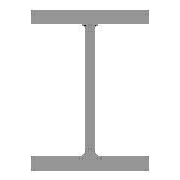
# Autodesk Inventor part: DIN 1025 - IPE 220-1497,05
Saved by Autodesk Inventor 2025 (Build 290162000, 162)
## iProperties
_CCFamilyMember: 80
_CCFamilyDisplayName: DIN 1025-5 IPE - Hot rolled I-beam IPE
_FrameMemberDoc: Frame Member File
_Version: 25.0.0
_GetPNFromCC: 1
Created: 2024-05-05
Part Number: DIN 1025 - IPE 220-1497,05
Material: Steel, Mild
Description: Hot rolled I-beam IPE
Document SubType Name: Modeling
Standard: DIN 1025
Designer: zulet
Standard Revision: 1994
Standards Organization: DIN
Language: en-US
Size Designation: IPE 220
Categories: <MemberInstance><Categories><Category DisplayName="Structural Shapes" InternalName="089c4875-fa83-4c05-b084-43b9cc11f5ed" Mnemonic="GRDR"><CategoryParameter DisplayName="Mass per Length Unit" InternalName="0bb95a10-148f-4027-a459-38d7b056702a" Mnemonic="shpmass"/><CategoryParameter DisplayName="Section Area" InternalName="1ff91680-64b0-4202-b9a3-7fd3f94bba3b" Mnemonic="secarea"/><CategoryParameter DisplayName="Radius of Gyration (x)" InternalName="25778675-03e9-40c1-b6a8-4a9ed693320d" Mnemonic="gyrradx"/><CategoryParameter DisplayName="Torsional Rigidity Modulus" InternalName="26c1ec35-5026-4c63-ad0a-751cf684a536" Mnemonic="torrigmod"/><CategoryParameter DisplayName="Distance of the Center of Gravity X-X" InternalName="26c9bdb8-9c79-4b4f-a92e-8e197583c9c4" Mnemonic="grcendistX"/><CategoryParameter DisplayName="Legacy Member ID" InternalName="340afe4f-75d7-48d3-ab7d-943f3c3da468" Mnemonic="LegacyMemberID"/><CategoryParameter DisplayName="Base Length" InternalName="42e34263-8f20-4d0e-ad48-bf1385b87c24" Mnemonic="shplen"/><CategoryParameter DisplayName="Moment of Inertia (y)" InternalName="4b9f58ea-bced-460e-81ea-3d29ca5a49e3" Mnemonic="inermomy"/><CategoryParameter DisplayName="Moment of Inertia (x)" InternalName="4cd780bc-73d7-43ac-917a-579e5cbd684d" Mnemonic="inermomx"/><CategoryParameter DisplayName="Custom Base Point" InternalName="4f1d1b73-316d-484b-a3df-9cbabb16eb77" Mnemonic="shpBasePoint"/><CategoryParameter DisplayName="Shape Height" InternalName="50274e7d-5ac0-4796-92cb-c59e54983c67" Mnemonic="shpheig"/><CategoryParameter DisplayName="Section Module (y)" InternalName="59eaa5e9-d227-48dc-b6c1-6920f96e0f95" Mnemonic="secmody"/><CategoryParameter DisplayName="Section Designation" InternalName="5a64d034-428d-49c8-ba32-7619764de20f" Mnemonic="shpdes"/><CategoryParameter DisplayName="Section Module (x)" InternalName="72cfad18-cf51-4ed4-aaa7-c6b224f8419f" Mnemonic="secmodx"/><CategoryParameter DisplayName="Torsional Section Modulus" InternalName="7c55a8dc-8844-49f9-a867-cc677b30ec9a" Mnemonic="torsecmod"/><CategoryParameter DisplayName="Shape Width" InternalName="7c717d54-a18f-4666-b4d4-573cce22c62c" Mnemonic="shpwdth"/><CategoryParameter DisplayName="Second Shape Thickness" InternalName="9251a8e1-85fd-4e47-af99-afdb762317d9" Mnemonic="shpthick2"/><CategoryParameter DisplayName="FG Authored" InternalName="9c666724-f362-4ea7-ac62-f6a007de5c69" Mnemonic="shpFGAuto"/><CategoryParameter DisplayName="Distance of the Center of Gravity Y-Y" InternalName="bcc4fb17-7af4-436a-8f8c-d0aa3b0248c5" Mnemonic="grcendistY"/><CategoryParameter DisplayName="Radius of Gyration (y)" InternalName="bfa18ebe-1636-4dbe-8d42-b263e0b73184" Mnemonic="gyrrady"/><CategoryParameter DisplayName="Shape Thickness" InternalName="d109cf76-8eb4-42fc-9800-4409734adc67" Mnemonic="shpthick"/><CategoryParameter DisplayName="Coefficient of Shear Displacement" InternalName="de4c90c6-aaa8-468f-a335-6737b311b5d3" Mnemonic="shdispc"/><Category DisplayName="I-Beams" InternalName="6918ea94-8af8-4304-ae03-7d2c1ce55d4b" Mnemonic="ISHP"><CategoryParameter DisplayName="Mass per Length Unit" InternalName="0dc32564-f4aa-4aa4-8c75-62cb498c92c3" Mnemonic="shpmass"/><CategoryParameter DisplayName="Radius of Gyration (y)" InternalName="0f8afd8f-b9f7-472e-8e75-9212891574fd" Mnemonic="gyrrady"/><CategoryParameter DisplayName="Second Shape Thickness" InternalName="391ebf09-f515-4c94-817f-86f5e53f4689" Mnemonic="shpthick2"/><CategoryParameter DisplayName="Moment of Inertia (x)" InternalName="a758f08a-3b45-4a09-8ee4-ba904e580c14" Mnemonic="inermomx"/><CategoryParameter DisplayName="Moment of Inertia (y)" InternalName="ae881498-39b5-464d-9622-212b1cfb5926" Mnemonic="inermomy"/><CategoryParameter DisplayName="Section Area" InternalName="bf9dd762-a4b6-4f54-802b-8b144141f7fb" Mnemonic="secarea"/><CategoryParameter DisplayName="Section Module (y)" InternalName="c0ad6f84-71f4-4f7a-a8c1-bbe4f36d703a" Mnemonic="secmody"/><CategoryParameter DisplayName="Shape Thickness" InternalName="c729d173-373e-41ba-bff7-d28a079d944c" Mnemonic="shpthick"/><CategoryParameter DisplayName="Radius of Gyration (x)" InternalName="db90017b-4fac-4daa-80b0-a7886743939d" Mnemonic="gyrradx"/><CategoryParameter DisplayName="Section Module (x)" InternalName="e71bf9c5-e82b-494f-914d-abe97254150e" Mnemonic="secmodx"/><CategoryParameter DisplayName="Shape Width" InternalName="f705f81c-b398-4253-aed1-763ae4858594" Mnemonic="shpwdth"/></Category></Category><Category DisplayName="DataType" InternalName="23b78d0f-2648-40c6-8793-ca6db495c9e8" Mnemonic="DATATYPE"><CategoryParameter DisplayName="DisplayName" InternalName="05415f3d-3907-474b-a020-eb9d644f4cf3" Mnemonic="DISPLAYNAME"/><CategoryParameter DisplayName="Standard" InternalName="0c0a119c-1e12-4c84-803f-101930972f5e" Mnemonic="STANDARD"/><CategoryParameter DisplayName="Description" InternalName="13903e3d-64b1-4950-80da-f627842ea37f" Mnemonic="DESCRIPTION"/><CategoryParameter DisplayName="Designation" InternalName="2675968c-4ce5-49e0-a4f5-552d29089031" Mnemonic="DESIGNATION"/><CategoryParameter DisplayName="Default Row" InternalName="2af9ec52-faaa-4026-b378-f9fa4afca842" Mnemonic="DEFAULTROW"/><CategoryParameter DisplayName="Folder Name" InternalName="3f06958e-8713-4116-9be7-ed6184ecc97b" Mnemonic="FOLDERNAME"/><CategoryParameter DisplayName="Revision Guid" InternalName="45a75005-10b1-4dfc-8d6d-dfe629f0b93c" Mnemonic="REVISIONGUID"/><CategoryParameter DisplayName="FileName" InternalName="8b46a4cc-9585-4fed-90c3-899f57e09a73" Mnemonic="FILENAME"/><CategoryParameter DisplayName="StdsOrg" InternalName="8f5914e1-4693-403f-8ab5-d37768198c9d" Mnemonic="STDSORG"/><CategoryParameter DisplayName="Family Version" InternalName="914462f6-6e19-4b14-ba84-155b9680b1d0" Mnemonic="FAMILYREVISION"/><CategoryParameter DisplayName="Standard Revision" InternalName="91d5a463-65c2-4fde-b823-3b7fea5e8e17" Mnemonic="STANDARDREVISION"/><CategoryParameter DisplayName="Member Revision" InternalName="a65d44b9-392f-4f4f-857b-e4b3d54996fe" Mnemonic="MEMBERREVISION"/><CategoryParameter DisplayName="ClipFormat" InternalName="bc51e27b-3422-4e78-93ef-cec197ddf230" Mnemonic="CLIPFORMAT"/><CategoryParameter DisplayName="Manufacturer" InternalName="cd6c7a72-a28a-4e50-99a9-2c7f4e13e5ad" Mnemonic="MANUFACTURER"/><CategoryParameter DisplayName="InternalName" InternalName="cf1d0246-76d9-4b4a-8305-fa0409afb5c1" Mnemonic="INTERNALNAME"/><CategoryParameter DisplayName="IsMetric" InternalName="e2385c5b-1ea4-4823-96a8-8de651266ec3" Mnemonic="ISMETRIC"/><Category DisplayName="Part" InternalName="c0e0b642-3bcb-4cc8-9e80-f96d35c4afa4" Mnemonic="PART"><CategoryParameter DisplayName="Part Number" InternalName="016b6077-bfbe-49bd-92c9-d8d59c39c941" Mnemonic="PARTNUMBER"/><CategoryParameter DisplayName="Stock Number" InternalName="4dba7c1c-e26c-444e-836c-b08b433409a8" Mnemonic="STOCKNUMBER"/><CategoryParameter DisplayName="Material Key" InternalName="5c9a8adb-dd2b-4535-b97f-0a94a95fe41f" Mnemonic="MATERIALKEY"/><CategoryParameter DisplayName="Material" InternalName="818a152a-d3c3-49ca-80ee-df7d91421b8e" Mnemonic="MATERIAL"/></Category></Category><Category DisplayName="LegacyMap" InternalName="cd87c42b-3e48-431e-b5c0-1cbeb14dfe77" Mnemonic="LEGACYMAP"><CategoryParameter DisplayName="unique DA member ID" InternalName="0918ad47-427f-4fed-ae26-24c81c58f590" Mnemonic="DACOOKIE"/><CategoryParameter DisplayName="Merge11 ID" InternalName="0ee8fb18-e2ed-4f39-96f6-1f4b5f50aa71" Mnemonic="MERGE11"/><CategoryParameter DisplayName="unique CC member ID" InternalName="5193edd4-b2b0-4ab4-9d54-de900eee34e0" Mnemonic="CCCOOKIE"/><CategoryParameter DisplayName="Split ID" InternalName="72b5c83c-be7f-45c4-ae51-9160ea6deb26" Mnemonic="SPLIT"/><CategoryParameter DisplayName="MemberID" InternalName="8e5e0294-fc51-4c8f-b3d7-003dc5ed94f6" Mnemonic="MEMBERID"/><CategoryParameter DisplayName="CatalogName" InternalName="d99d1e27-aa94-4de2-af4c-c348882a6f4f" Mnemonic="CATALOGNAME"/><CategoryParameter DisplayName="FamilyNumber" InternalName="e705e1f4-09cb-413e-91f9-551b4188271e" Mnemonic="FAMILYNUMBER"/></Category></Categories><FamilyTemplate Id="D1025_2"><FamilyTemplateParameters><FamilyTemplateParameter ObjectType="kUserParameterObject" ValueType="xs:double" Id="1" ObjectReferenceKey="ParH"/><FamilyTemplateParameter ObjectType="kUserParameterObject" ValueType="xs:double" Id="2" ObjectReferenceKey="b"/><FamilyTemplateParameter ObjectType="kUserParameterObject" ValueType="xs:double" Id="3" ObjectReferenceKey="B_L"/><FamilyTemplateParameter ObjectType="kUserParameterObject" ValueType="xs:double" Id="4" ObjectReferenceKey="t1"/><FamilyTemplateParameter ObjectType="kUserParameterObject" ValueType="xs:double" Id="5" ObjectReferenceKey="t2"/><FamilyTemplateParameter ObjectType="kUserParameterObject" ValueType="xs:double" Id="6" ObjectReferenceKey="R1"/><FamilyTemplateParameter ObjectType="kPropertyObject" ValueType="xs:string" Id="100" ObjectReferenceKey="{32853F0F-3444-11d1-9E93-0060B03C1CA6}" SubObjectId="52"/><FamilyTemplateParameter ObjectType="kPropertyObject" ValueType="xs:string" Id="105" ObjectReferenceKey="{32853F0F-3444-11d1-9E93-0060B03C1CA6}" SubObjectId="5"/><FamilyTemplateParameter ObjectType="kPartComponentDefinitionObject" ValueType="xs:string" Id="110" SubObjectId="Material"/><FamilyTemplateParameter ObjectType="kPropertyObject" ValueType="xs:string" Id="112" ObjectReferenceKey="{32853F0F-3444-11d1-9E93-0060B03C1CA6}" SubObjectId="55"/></FamilyTemplateParameters></FamilyTemplate><CategoryParameterMap><ParamToTemplateMap><ParamToTemplate CategoryParameter="//CategoryParameter[@InternalName='05415f3d-3907-474b-a020-eb9d644f4cf3']" ConstantValue="DIN 1025-5 IPE"/><ParamToTemplate CategoryParameter="//CategoryParameter[@InternalName='cf1d0246-76d9-4b4a-8305-fa0409afb5c1']" ConstantValue="11DEA241-3E29-4894-9654-6C8D07453054"/><ParamToTemplate CategoryParameter="//CategoryParameter[@InternalName='3f06958e-8713-4116-9be7-ed6184ecc97b']" ConstantValue="DIN 1025 IPE"/><ParamToTemplate CategoryParameter="//CategoryParameter[@InternalName='914462f6-6e19-4b14-ba84-155b9680b1d0']" ConstantValue="10"/><ParamToTemplate CategoryParameter="//CategoryParameter[@InternalName='bc51e27b-3422-4e78-93ef-cec197ddf230']" ConstantValue="CF_INVENTOR.STDPARTS"/><ParamToTemplate CategoryParameter="//CategoryParameter[@InternalName='e2385c5b-1ea4-4823-96a8-8de651266ec3']" ConstantValue="true"/><ParamToTemplate CategoryParameter="//CategoryParameter[@InternalName='13903e3d-64b1-4950-80da-f627842ea37f']" ConstantValue="Hot rolled I-beam IPE"/><ParamToTemplate CategoryParameter="//CategoryParameter[@InternalName='8f5914e1-4693-403f-8ab5-d37768198c9d']" ConstantValue="DIN"/><ParamToTemplate CategoryParameter="//CategoryParameter[@InternalName='0c0a119c-1e12-4c84-803f-101930972f5e']" ConstantValue="DIN 1025"/><ParamToTemplate CategoryParameter="//CategoryParameter[@InternalName='cd6c7a72-a28a-4e50-99a9-2c7f4e13e5ad']" TemplateParameter="104"/><ParamToTemplate CategoryParameter="//CategoryParameter[@InternalName='91d5a463-65c2-4fde-b823-3b7fea5e8e17']" ConstantValue="1994"/><ParamToTemplate CategoryParameter="//CategoryParameter[@InternalName='45a75005-10b1-4dfc-8d6d-dfe629f0b93c']" ConstantValue="b36a5bb9-0290-4eb4-bba2-e462c37a096a"/><ParamToTemplate CategoryParameter="//CategoryParameter[@InternalName='2af9ec52-faaa-4026-b378-f9fa4afca842']" ConstantValue="10"/><ParamToTemplate CategoryParameter="//CategoryParameter[@InternalName='9c666724-f362-4ea7-ac62-f6a007de5c69']" ConstantValue="1"/><ParamToTemplate CategoryParameter="//CategoryParameter[@InternalName='8b46a4cc-9585-4fed-90c3-899f57e09a73']" ConstantValue="DIN 1025 - IPE 360-1"/><ParamToTemplate CategoryParameter="//CategoryParameter[@InternalName='a65d44b9-392f-4f4f-857b-e4b3d54996fe']" ConstantValue="2F7BE790-9201-4313-A6B9-FAB6FCE7215E"/><ParamToTemplate CategoryParameter="//CategoryParameter[@InternalName='a758f08a-3b45-4a09-8ee4-ba904e580c14']" ConstantValue="1.627e+008"/><ParamToTemplate CategoryParameter="//CategoryParameter[@InternalName='ae881498-39b5-464d-9622-212b1cfb5926']" ConstantValue="1.04e+007"/><ParamToTemplate CategoryParameter="//CategoryParameter[@InternalName='e71bf9c5-e82b-494f-914d-abe97254150e']" ConstantValue="904000"/><ParamToTemplate CategoryParameter="//CategoryParameter[@InternalName='c0ad6f84-71f4-4f7a-a8c1-bbe4f36d703a']" ConstantValue="123000"/><ParamToTemplate CategoryParameter="//CategoryParameter[@InternalName='bf9dd762-a4b6-4f54-802b-8b144141f7fb']" ConstantValue="7270"/><ParamToTemplate CategoryParameter="//CategoryParameter[@InternalName='7c55a8dc-8844-49f9-a867-cc677b30ec9a']" ConstantValue="29381,034"/><ParamToTemplate CategoryParameter="//CategoryParameter[@InternalName='26c1ec35-5026-4c63-ad0a-751cf684a536']" ConstantValue="373139,13"/><ParamToTemplate CategoryParameter="//CategoryParameter[@InternalName='de4c90c6-aaa8-468f-a335-6737b311b5d3']" ConstantValue="2,1"/><ParamToTemplate CategoryParameter="//CategoryParameter[@InternalName='db90017b-4fac-4daa-80b0-a7886743939d']" ConstantValue="150"/><ParamToTemplate CategoryParameter="//CategoryParameter[@InternalName='0f8afd8f-b9f7-472e-8e75-9212891574fd']" ConstantValue="37,9"/><ParamToTemplate CategoryParameter="//CategoryParameter[@InternalName='0918ad47-427f-4fed-ae26-24c81c58f590']" ConstantValue="*DIN~D1025_5~IPE 360-25000*"/><ParamToTemplate CategoryParameter="//CategoryParameter[@InternalName='0ee8fb18-e2ed-4f39-96f6-1f4b5f50aa71']" ConstantValue="^38b60987-b6a5-40f3-bbfa-fc2af2db0cf9#13^5B1291D4-26CA-46F0-A3B1-56EC9DD4A035#130^"/><ParamToTemplate CategoryParameter="//CategoryParameter[@InternalName='42e34263-8f20-4d0e-ad48-bf1385b87c24']" TemplateParameter="3"/><ParamToTemplate CategoryParameter="//CategoryParameter[@InternalName='2675968c-4ce5-49e0-a4f5-552d29089031']" TemplateParameter="100"/><ParamToTemplate CategoryParameter="//CategoryParameter[@InternalName='818a152a-d3c3-49ca-80ee-df7d91421b8e']" TemplateParameter="110"/><ParamToTemplate CategoryParameter="//CategoryParameter[@InternalName='016b6077-bfbe-49bd-92c9-d8d59c39c941']" TemplateParameter="105"/><ParamToTemplate CategoryParameter="//CategoryParameter[@InternalName='50274e7d-5ac0-4796-92cb-c59e54983c67']" TemplateParameter="1"/><ParamToTemplate CategoryParameter="//CategoryParameter[@InternalName='4dba7c1c-e26c-444e-836c-b08b433409a8']" TemplateParameter="112"/><ParamToTemplate CategoryParameter="//CategoryParameter[@InternalName='f705f81c-b398-4253-aed1-763ae4858594']" TemplateParameter="2"/><ParamToTemplate CategoryParameter="//CategoryParameter[@InternalName='c729d173-373e-41ba-bff7-d28a079d944c']" TemplateParameter="4"/></ParamToTemplateMap></CategoryParameterMap></MemberInstance>
Stock Number: IPE 220
Density: 7.85 g/cm^3
Appearance: Semi-Polished
IsCustomPart: 1
G_L: 1497,050 mm
G_W: 110,000 mm
G_H: 220,000 mm
+E306E2F0-DEFC-4B6E-B958-F0CDA3C58A72+CUTDETAIL1: Miter 45,00 deg
+04264D6A-114A-40A8-9F54-E6A20931D243+CUTDETAIL2: Miter 45,00 deg
+CD89E8C5-F45F-4157-B7D0-56B8621B9B92+CUTDETAIL3: Notch
+736B08D9-697D-49D8-92AA-A86A60E3E6FB+CUTDETAIL4: Notch
Author: zulet
Autodesk Inventor part; units mm, degrees
ref_plane "YZ Plane" through (0, 0, 0) normal (1, 0, 0) x (0, 1, 0)
ref_plane "XZ Plane" through (0, 0, 0) normal (0, 1, 0) x (-1, 0, 0)
ref_plane "XY Plane" through (0, 0, 0) normal (0, 0, 1) x (1, 0, 0)
ref_plane "Start plane" through (0, 0, 0) normal (0, 0, 1) x (1, 0, 0)
ref_plane "End plane" through (0, 0, 1497.05) normal (0, 0, 1) x (1, 0, 0)
sketch "Sketch2" plane through (0, 0, 0) normal (0, 0, 1) x (1, 0, 0)
  line L0 (-55, 100.8) -> (-14.95, 100.8)
  line L1 (-55, 110) -> (-55, 100.8)
  line L2 (55, 110) -> (-55, 110)
  line L3 (55, 100.8) -> (55, 110)
  line L4 (14.95, 100.8) -> (55, 100.8)
  line L5 (2.95, -88.8) -> (2.95, 88.8)
  line L6 (55, -100.8) -> (14.95, -100.8)
  line L7 (55, -110) -> (55, -100.8)
  line L8 (-55, -100.8) -> (-55, -110)
  line L9 (-14.95, -100.8) -> (-55, -100.8)
  line L10 (-2.95, 88.8) -> (-2.95, -88.8)
  line L11 (0, -154) -> (0, 154) construction
  line L12 (-2.95, -100.8) -> (2.95, -100.8) construction
  arc A0 (-14.95, -100.8) -> (-2.95, -88.8) centre (-14.95, -88.8) ccw
  arc A1 (-2.95, 88.8) -> (-14.95, 100.8) centre (-14.95, 88.8) ccw
  arc A2 (14.95, 100.8) -> (2.95, 88.8) centre (14.95, 88.8) ccw
  arc A3 (2.95, -88.8) -> (14.95, -100.8) centre (14.95, -88.8) ccw
  line L13 (-77, 0) -> (77, 0) construction
  line L14 (-55, -110) -> (55, -110)
  point P0 (-2.95, 100.8)
  point P1 (2.95, 100.8)
  point P2 (0, 0)
  point P3 (0, -100.8)
  point P4 (0, 0)
  dimension "d1" = 220
  dimension "d3" = 9.2
  dimension "d5" = 5.9
  dimension "d7" = 110
  dimension "d13" = 12
  dimension "d14" = 110
  dimension "d15" = 55
  constraints: 26 end point, 9 point on line, 8 point on circle, 8 tangent, 6 vertical, 5 collinear, 5 horizontal, 4 centre point, 3 equal radius, 2 midpoint, 1 parallel, 1 perpendicular
  measures "d1" distance of L7.start L2.start
  measures "d3" distance of L1.start L0.start
  measures "d5" distance of point (-2.95, 100.8) point (2.95, 100.8)
  measures "d7" distance of L2.start L1.start
  measures "d13" radius of A0
  measures "d14" distance between parallel lines of L2 L13
  measures "d15" distance between parallel lines of L7 L11
extrude "Body" add sketch "Sketch2" along normal up to surface (1497.05 mm away) from surface at 0
sketch "Sketch3" plane through (0, 0, 0) normal (0, 0, 1) x (1, 0, 0)
  line L0 (0, 0) -> (10, 0)
ref_plane "Work Plane3" through (0, 0, 0) normal (0, -1, 0) x (1, 0, 0)
ref_plane "Work Plane4" through (55, 0, -55) normal (-0.7071068, 0, -0.7071068) x (-0.7071068, 0, 0.7071068)
split "Split1" plane through (55, 0, -55) removes the side toward (-0.7071068, 0, -0.7071068)
ref_plane "Work Plane5" through (-55, 0, -55) normal (0.7071068, 0, -0.7071068) x (-0.7071068, 0, -0.7071068)
split "Split2" plane through (-55, 0, -55) removes the side toward (0.7071068, 0, -0.7071068)
ref_plane "Work Plane6" through (0, 0, 1500) normal (1, 0, 0) x (0, 0, -1)
ref_plane "Work Plane7" through (1555, 0, 1555) normal (0.7071068, 0, -0.7071068) x (-0.7071068, 0, -0.7071068)
ref_plane "Work Plane8" through (750, 0, 1500) normal (1, 0, 0) x (0, 0, -1)
ref_plane "Work Plane9" through (0, 0, 1500) normal (-1, 0, 0) x (0, 0, 1)
ref_plane "Work Plane10" through (-1500, 0, 1500) normal (-1, 0, 0) x (0, 0, 1)
ref_plane "Work Plane11" through (-750, 0, 1500) normal (-1, 0, 0) x (0, 0, 1)
sketch "Sketch5" plane through (750, 0, 1500) normal (1, 0, 0) x (0, 0, -1)
  line L0 (-55, 100.8) -> (-14.95, 100.8)
  arc A0 (-2.95, 88.8) -> (-14.95, 100.8) centre (-14.95, 88.8) ccw
  line L1 (-2.95, 88.8) -> (-2.95, -88.8)
  arc A1 (-14.95, -100.8) -> (-2.95, -88.8) centre (-14.95, -88.8) ccw
  line L2 (-14.95, -100.8) -> (-55, -100.8)
  line L3 (-55, -100.8) -> (-55, -110)
  line L4 (-55, -110) -> (55, -110)
  line L5 (55, -110) -> (55, -100.8)
  line L6 (55, -100.8) -> (14.95, -100.8)
  arc A2 (2.95, -88.8) -> (14.95, -100.8) centre (14.95, -88.8) ccw
  line L7 (2.95, -88.8) -> (2.95, 88.8)
  arc A3 (14.95, 100.8) -> (2.95, 88.8) centre (14.95, 88.8) ccw
  line L8 (14.95, 100.8) -> (55, 100.8)
  line L9 (55, 100.8) -> (55, 110)
  line L10 (55, 110) -> (-55, 110)
  line L11 (-55, 110) -> (-55, 100.8)
  constraints: 24 end point, 8 point on circle, 4 centre point
extrude "Extrusion2" add sketch "Sketch5" along normal up to surface from surface at -750 separate body surface through (1555, 0, 1555) normal (0.7071068, 0, -0.7071068)
combine bodies "Combine1" operation type subtract main body 1 bodies to subtract 2
sketch "Sketch6" plane through (-750, 0, 1500) normal (-1, 0, 0) x (0, 0, 1)
  line L0 (-55, 100.8) -> (-14.95, 100.8)
  arc A0 (-2.95, 88.8) -> (-14.95, 100.8) centre (-14.95, 88.8) ccw
  line L1 (-2.95, 88.8) -> (-2.95, -88.8)
  arc A1 (-14.95, -100.8) -> (-2.95, -88.8) centre (-14.95, -88.8) ccw
  line L2 (-14.95, -100.8) -> (-55, -100.8)
  line L3 (-55, -100.8) -> (-55, -110)
  line L4 (-55, -110) -> (55, -110)
  line L5 (55, -110) -> (55, -100.8)
  line L6 (55, -100.8) -> (14.95, -100.8)
  arc A2 (2.95, -88.8) -> (14.95, -100.8) centre (14.95, -88.8) ccw
  line L7 (2.95, -88.8) -> (2.95, 88.8)
  arc A3 (14.95, 100.8) -> (2.95, 88.8) centre (14.95, 88.8) ccw
  line L8 (14.95, 100.8) -> (55, 100.8)
  line L9 (55, 100.8) -> (55, 110)
  line L10 (55, 110) -> (-55, 110)
  line L11 (-55, 110) -> (-55, 100.8)
  constraints: 24 end point, 8 point on circle, 4 centre point
extrude "Extrusion3" add sketch "Sketch6" along normal up to surface (1500 mm away) from surface at -750 separate body
combine bodies "Combine2" operation type subtract main body 1 bodies to subtract 3
sketch "Sketch4" plane through (0, 0, 0) normal (0, -1, 0) x (1, 0, 0)
  line L0 (-2, 0) -> (12, 0) projected
  line L1 (-2, 1497.05) -> (12, 1497.05) projected
  dimension "d19" = 1497.05
  measures "d19" distance between parallel lines of L0 L1
equation "\"d1\" = ParH"
equation "\"d3\" = t2"
equation "\"d5\" = t1"
equation "\"d7\" = b"
equation "\"d13\" = R1"
equation "\"d14\" = 0.5 * d1"
equation "\"d15\" = 0.5 * d7"
equation "\"d8\" = G_L"
equation "\"b\" = 110"
equation "\"ParH\" = 220"
equation "\"R1\" = 12"
equation "\"G_L\" = 1497.05"
equation "\"t1\" = 5.9"
equation "\"t2\" = 9.2"
equation "\"G_OFFSET_START\" = 0"
equation "\"G_OFFSET_END\" = -2.95"
equation "\"d17\" = G_OFFSET_END + B_L"
equation "\"B_L\" = 1500"
body "Solid1"
body "Solid8"
body "Solid9"
